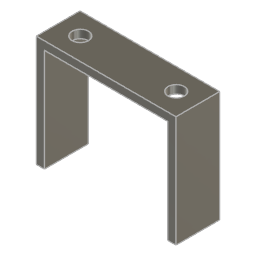
protege motores (Autodesk Fusion 360 design; units mm, degrees)
Autodesk Fusion 360 part; units mm, degrees
sketch "Boceto5" plane through (-11.25, 0, 0) normal (-1, 0, 0) x (0, -1, 0)
sketch "Boceto8" plane through (12.75, 0, 0) normal (1, 0, 0) x (0, 1, 0)
  line L0 (-15.65, 0) -> (-25.65, 0)
  line L1 (-25.65, 0) -> (-25.65, -18.8)
  line L2 (-25.65, -18.8) -> (-15.65, -18.8)
  line L3 (-15.65, -18.8) -> (-15.65, 0)
  line L4 (-25.65, 0) -> (-25.65, 1.5)
  line L5 (-25.65, 1.5) -> (-15.65, 1.5)
  line L6 (-15.65, 1.5) -> (-15.65, 0)
  dimension "d15" = 1.5
  constraint coincident L0.end L1.start
  constraint perpendicular L0 L4
  constraint perpendicular L3 L5
  constraint coincident L0.start L3.end
  constraint perpendicular L0 L6
  measures "d15" distance of L0.end L4.end
sketch "Boceto10" plane through (0, -25.65, 0) normal (0, -1, 0) x (1, 0, 0)
  line L0 (12.75, 0) -> (12.75, 1.5)
  line L1 (12.75, 1.5) -> (-12.75, 1.5)
  line L2 (-12.75, 1.5) -> (-12.75, 0)
  line L3 (-12.75, 0) -> (12.75, 0)
  line L4 (-12.75, 0) -> (-12.75, 1.5)
  line L5 (12.75, 1.5) -> (-12.75, 1.5)
  line L6 (12.75, 1.5) -> (12.75, 0)
  line L7 (11.25, -18.8) -> (12.75, 0)
  line L8 (11.25, -18.8) -> (12.75, 0)
  line L9 (-12.75, 0) -> (12.75, 0)
  line L10 (-11.25, -18.8) -> (-12.75, 0)
  line L11 (-11.25, -18.8) -> (-12.75, 0)
  constraint coincident L2.end L3.start
  constraint coincident L1.end L2.start
  constraint coincident L0.end L1.start
  constraint coincident L0.start L3.end
sketch "Boceto11" plane through (11.25, 0, 0) normal (1, 0, 0) x (0, 1, 0)
  line L0 (-25.65, -10.05) -> (-25.65, -18.8)
  line L1 (-25.65, -18.8) -> (7.2, -18.8)
  line L2 (7.2, -18.8) -> (7.2, 0)
  line L3 (7.2, 0) -> (-25.65, 0)
  line L4 (-25.65, 0) -> (-25.65, -10.05)
  line L5 (-24.65, 0) -> (-16.65, 0)
  line L6 (-24.65, 0) -> (-24.65, -18.8)
  line L7 (-16.65, 0) -> (-16.65, -18.8)
  dimension "d22" = 1
  dimension "d23" = 8
  constraint coincident L1 L6.end
  constraint perpendicular L1 L6
  constraint coincident L1 L7.end
  constraint perpendicular L1 L7
  measures "d22" distance of L3.end L5.start
  measures "d23" distance of L5.start L5.end
extrude "Extruir7" add sketch "Boceto11" along normal blind 1.5 contours L1 L3 L5 L6 L7
sketch "Boceto12" plane through (12.75, 0, 0) normal (1, 0, 0) x (0, 1, 0)
  line L0 (-24.65, 0) -> (-24.65, -18.8)
  line L1 (-24.65, -18.8) -> (-16.65, -18.8)
  line L2 (-16.65, -18.8) -> (-16.65, 0)
  line L3 (-16.65, 0) -> (-24.65, 0)
  line L4 (-24.65, 0) -> (-24.65, 1.5)
  line L5 (-16.65, 0) -> (-16.65, 1.5)
  line L6 (-16.65, 1.5) -> (-24.65, 1.5)
  dimension "d26" = 1.5
  dimension "d27" = 1.5
  constraint coincident L0.start L3.end
  constraint perpendicular L3 L4
  constraint coincident L2.end L3.start
  constraint perpendicular L3 L5
  measures "d26" distance of L0.start L4.end
  measures "d27" distance of L2.end L5.end
extrude "Extruir8" add sketch "Boceto12" against normal blind 25.5 contours L3 L4 L5 L6
sketch "Boceto13" plane through (0, 0, 0) normal (0, 0, -1) x (1, 0, 0)
  line L0 (11.25, 16.65) -> (11.25, 24.65)
  line L1 (11.25, 24.65) -> (-12.75, 24.65)
  line L2 (-12.75, 24.65) -> (-12.75, 16.65)
  line L3 (-12.75, 16.65) -> (11.25, 16.65)
  line L4 (-12.75, 24.65) -> (-11.25, 24.65)
  line L5 (-12.75, 24.65) -> (-12.75, 16.65)
  line L6 (-12.75, 16.65) -> (-11.25, 16.65)
  line L7 (-11.25, 16.65) -> (-11.25, 24.65)
  dimension "d30" = 1.5
  dimension "d31" = 1.5
  constraint coincident L1.end L2.start
  constraint perpendicular L2 L4
  constraint coincident L2.end L3.start
  constraint perpendicular L2 L6
  measures "d30" distance of L1.end L4.end
  measures "d31" distance of L2.end L6.end
extrude "Extruir9" add sketch "Boceto13" along normal blind 18.8 contours L1 L2 L3 L4 L5 L6 L7
sketch "Boceto14" plane through (0, 0, -18.8) normal (0, 0, -1) x (1, 0, 0)
  line L0 (-7.25, -11.2) -> (7.25, -11.2)
  arc A0 (7.25, -11.2) -> (11.25, -7.2) centre (7.25, -7.2) ccw
  line L1 (11.25, -7.2) -> (11.25, 25.65)
  line L2 (11.25, 25.65) -> (7.0711, 25.65)
  line L3 (7.0711, 25.65) -> (7.0711, 37.15)
  line L4 (7.0711, 37.15) -> (-7.0711, 37.15)
  line L5 (-7.0711, 37.15) -> (-7.0711, 25.65)
  line L6 (-7.0711, 25.65) -> (-11.25, 25.65)
  line L7 (-11.25, 25.65) -> (-11.25, -7.2)
  arc A1 (-11.25, -7.2) -> (-7.25, -11.2) centre (-7.25, -7.2) ccw
  circle A2 centre (8.75, 20.6) radius 1.5
  circle A3 centre (-8.75, 20.6) radius 1.5
  circle A4 centre (0, 0) radius 2.7
  line L8 (-2.5, 31.15) -> (-2.5, 32.8199)
  line L9 (-2.5, 32.8199) -> (2.5, 32.8199)
  line L10 (2.5, 32.8199) -> (2.5, 31.15)
  line L11 (2.5, 31.15) -> (-2.5, 31.15)
  circle A5 centre (8.75, 20.6) radius 1.5
  constraint concentric A2 A5
extrude "Extruir10" cut sketch "Boceto14" against normal blind 25 contours A2 A5 | A3
